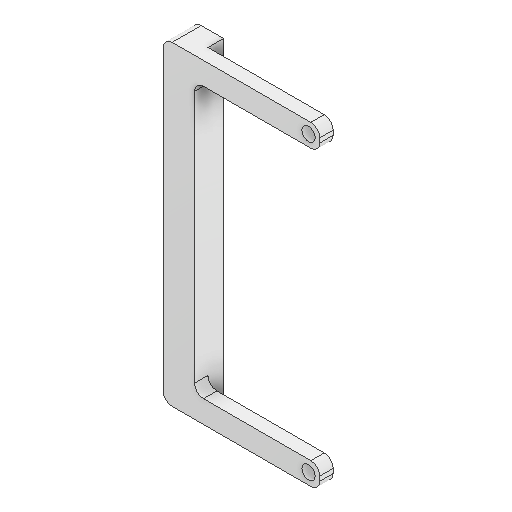
# Autodesk Inventor part: Display_Hilder
Saved by Autodesk Inventor 2025.2 (Build 292293000, 293)
## iProperties
Created: 2025-03-12
Part Number: Display_Hilder
Material: PC/ABS Plastic
Document SubType Name: Modeling
Designer: ahorat
Density: 1.1 g/cm^3
Appearance: Smooth - White
Mass: 4.38793 g
Surface Area: 28.853 cm^2
Volume: 3.98903 cm^3
Author: ahorat
Autodesk Inventor part; units mm, degrees
ref_plane "YZ Plane" through (0, 0, 0) normal (1, 0, 0) x (0, 1, 0)
ref_plane "XZ Plane" through (0, 0, 0) normal (0, 1, 0) x (-1, 0, 0)
ref_plane "XY Plane" through (0, 0, 0) normal (0, 0, 1) x (1, 0, 0)
sketch "Sketch1" plane through (0, 0, 0) normal (0, 0, 1) x (1, 0, 0)
  line L0 (31.5, 30.25) -> (31.5, 35.25)
  line L1 (31.5, 35.25) -> (-3.5, 35.25)
  line L2 (-3.5, 35.25) -> (-3.5, 0)
  line L3 (-3.5, 0) -> (3.5, 0)
  line L4 (3.5, 0) -> (3.5, 30.25)
  line L5 (3.5, 30.25) -> (31.5, 30.25)
  point P0 (0, 0)
  point P1 (0, 0)
  point P2 (31.5, 32.75)
  dimension "d0" = 7
  dimension "d2" = 5
  dimension "d3" = 35
  dimension "d4" = 32.75
  constraints: 12 end point, 5 perpendicular, 2 midpoint, 1 coincident, 1 vertical
  measures "d0" distance of L2.end L3.end
  measures "d2" distance of L0.start L0.end
  measures "d3" distance of L0.end L1.end
  measures "d4" distance from line of L3 point (31.5, 32.75)
extrude "Extrusion1" add sketch "Sketch1" along normal blind 3
mirror "Mirror1" about plane through (0, 0, 0) normal (0, 1, 0) of "Extrusion1"
sketch "Sketch2" plane through (0, 0, 0) normal (0, 0, -1) x (-1, 0, 0)
  line L0 (-31.5, -35.25) -> (3.5, -35.25) projected
  line L1 (-31.5, 35.25) -> (3.5, 35.25) projected
  line L2 (3.5, -35.25) -> (-3.5, -35.25)
  line L3 (-3.5, -35.25) -> (-3.5, 35.25)
  line L4 (-3.5, 35.25) -> (3.5, 35.25)
  line L5 (3.5, 35.25) -> (3.5, -35.25)
  line L6 (-3.5, 30.25) -> (-3.5, -30.25) projected
  point P0 (0, 0)
  point P1 (-3.5, 0)
  point P2 (3.5, 35.25)
  point P3 (-3.5, -35.25)
  constraints: 8 end point, 2 midpoint, 2 parallel, 1 horizontal, 1 perpendicular, 1 point on line
extrude "Extrusion2" add sketch "Sketch2" along normal blind 3.5
sketch "Sketch3" plane through (0, 0, 3) normal (0, 0, 1) x (1, 0, 0)
  line L0 (29, 32.75) -> (29, -32.75)
  line L1 (31.5, 30.25) -> (31.5, 35.25) projected
  point P0 (0, 0)
  point P1 (29, 0)
  dimension "d16" = 65.5
  dimension "d18" = 2.5
  constraints: 2 end point, 1 horizontal alignment, 1 midpoint, 1 vertical
  measures "d16" distance of L0.start L0.end
  measures "d18" distance from line of L1 L0.start
hole "Hole1" at (29, -32.75, 3) at (29, 32.75, 3) direction (0, 0, -1) diameter 3 end through all
fillet "Fillet1" radius 2 8 edges at (31.5, -35.25, 1.5) (31.5, -30.25, 1.5) (31.5, 30.25, 1.5) (31.5, 35.25, 1.5) (-3.5, -35.25, -0.25) (-3.5, 35.25, -0.25) (3.5, -30.25, 1.5) (3.5, 30.25, 1.5)
body "Solid1"
